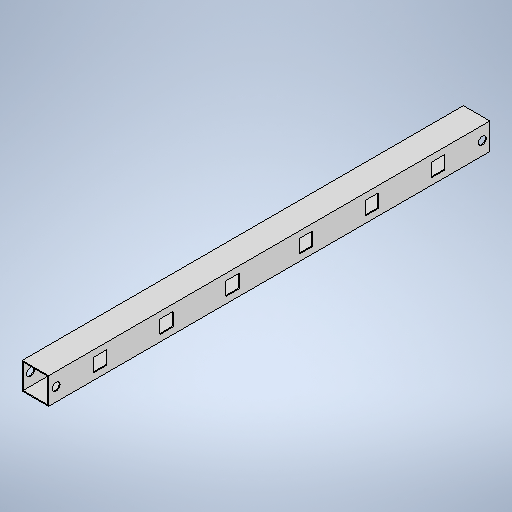
# Autodesk Inventor part: TZS 1761 FDS 1200x50 central way
Saved by Autodesk Inventor 2025.1 (Build 291241020, 241B)
## iProperties
Created: 2025-06-24
Part Number: TZS 1761 FDS 1200x50 central way
Material: Stainless Steel
Document SubType Name: Modeling
Designer: user
Mass: 1762.25 g
Surface Area: 2283.33 cm^2
Volume: 220.281 cm^3
Density: 8 g/cm^3
Sheet Metal Rule: AISI304 2mm Die16
Sheet Metal Width: 0.000 mm
Sheet Metal Length: 0.000 mm
Sheet Metal Area: 0.000 mm^2
Appearance: Default
Author: user
Autodesk Inventor part; units mm, degrees
ref_plane "YZ Plane" through (0, 0, 0) normal (1, 0, 0) x (0, 1, 0)
ref_plane "XZ Plane" through (0, 0, 0) normal (0, 1, 0) x (-1, 0, 0)
ref_plane "XY Plane" through (0, 0, 0) normal (0, 0, 1) x (1, 0, 0)
sketch "Sketch9" plane through (0, 0, 0) normal (0, 1, 0) x (-1, 0, 0)
  line L0 (30, 30) -> (-30, 30)
  line L1 (-30, 30) -> (-30, -30)
  line L2 (-30, -30) -> (30, -30)
  line L3 (30, -30) -> (30, 30)
  line L4 (30, 30) -> (-30, -30) construction
  line L5 (-30, 30) -> (30, -30) construction
  line L6 (-28, 28) -> (28, 28)
  line L7 (28, 28) -> (28, -28)
  line L8 (28, -28) -> (-28, -28)
  line L9 (-28, -28) -> (-28, 28)
  point P0 (0, 0)
  dimension "d172" = 60
  dimension "d173" = 60
  dimension "d174" = 2
  constraints: 20 end point, 4 parallel, 2 midpoint, 2 perpendicular, 1 horizontal, 3 other
  measures "d172" distance of L2.end L1.end
  measures "d173" distance of L0.end L1.end
  measures "d174" distance between parallel lines of L0 L6
extrude "Extrusion3" add sketch "Sketch9" against normal blind 500
sketch "Sketch10" plane through (0, 0, 0) normal (1, 0, 0) x (0, 1, 0)
  line L0 (0, 30) -> (0, -30) construction
  line L1 (0, 30) -> (-500, 30) construction
  line L2 (-500, -30) -> (-500, 30) construction
  line L3 (0, -30) -> (-500, -30) construction
  line L4 (-98.25, 15.25) -> (-67.75, 15.25)
  line L5 (-67.75, 15.25) -> (-67.75, -15.25)
  line L6 (-67.75, -15.25) -> (-98.25, -15.25)
  line L7 (-98.25, -15.25) -> (-98.25, 15.25)
  line L8 (-98.25, 15.25) -> (-67.75, -15.25) construction
  line L9 (-67.75, 15.25) -> (-98.25, -15.25) construction
  line L10 (-248.25, 15.25) -> (-217.75, 15.25)
  line L11 (-217.75, 15.25) -> (-217.75, -15.25)
  line L12 (-217.75, -15.25) -> (-248.25, -15.25)
  line L13 (-248.25, -15.25) -> (-248.25, 15.25)
  line L14 (-248.25, 15.25) -> (-217.75, -15.25) construction
  line L15 (-217.75, 15.25) -> (-248.25, -15.25) construction
  line L16 (-398.25, 15.25) -> (-367.75, 15.25)
  line L17 (-367.75, 15.25) -> (-367.75, -15.25)
  line L18 (-367.75, -15.25) -> (-398.25, -15.25)
  line L19 (-398.25, -15.25) -> (-398.25, 15.25)
  line L20 (-398.25, 15.25) -> (-367.75, -15.25) construction
  line L21 (-367.75, 15.25) -> (-398.25, -15.25) construction
  circle A0 centre (-483, 0) radius 9
  line L22 (0, 0) -> (47, 0)
  point P0 (-83, 0)
  point P1 (-233, 0)
  point P2 (-383, 0)
  dimension "d177" = 30.5
  dimension "d178" = 30.5
  dimension "d181" = 47
  dimension "d182" = 130
  dimension "d183" = 280
  dimension "d184" = 430
  dimension "d185" = 530
  dimension "d186" = 18
  constraints: 38 end point, 7 midpoint, 6 parallel, 4 horizontal, 4 horizontal alignment, 3 equal length, 3 perpendicular, 1 centre point, 1 point on line
  measures "d177" distance of L4.start L4.end
  measures "d178" distance of L4.end L5.end
  measures "d181" distance of L22.start L22.end
  measures "d182" distance of point (-83, 0) L22.end
  measures "d183" distance of point (-233, 0) L22.end
  measures "d184" distance of L22.end point (-383, 0)
  measures "d185" distance of L22.end A0.centre
  measures "d186" diameter of A0
extrude "Extrusion4" cut sketch "Sketch10" along normal through all both and the other way through all
fillet "Fillet1" radius 2 24 edges at (29, -367.75, -15.25) (29, -367.75, 15.25) (29, -398.25, 15.25) (29, -398.25, -15.25) (29, -248.25, -15.25) (29, -248.25, 15.25) (29, -217.75, 15.25) (29, -217.75, -15.25) (29, -98.25, 15.25) (29, -67.75, 15.25) (29, -67.75, -15.25) (29, -98.25, -15.25) (-29, -98.25, 15.25) (-29, -67.75, 15.25) (-29, -67.75, -15.25) (-29, -98.25, -15.25) (-29, -217.75, 15.25) (-29, -248.25, 15.25) (-29, -248.25, -15.25) (-29, -217.75, -15.25) (-29, -367.75, 15.25) (-29, -398.25, 15.25) (-29, -367.75, -15.25) (-29, -398.25, -15.25)
mirror "Mirror1" about plane through (0, 0, 0) normal (0, 1, 0) of "Extrusion3", "Extrusion4", "Fillet1"
sketch "Sketch14" plane through (30, -500, -30) normal (0, 0, -1) x (-1, 0, 0)
  line L0 (57, 527) -> (3, 527)
  line L1 (3, 527) -> (3, 473)
  line L2 (3, 473) -> (57, 473)
  line L3 (57, 473) -> (57, 527)
  line L4 (57, 527) -> (3, 473) construction
  line L5 (3, 527) -> (57, 473) construction
  point P0 (30, 500)
  dimension "d188" = 54
  constraints: 12 end point, 2 midpoint, 2 parallel, 2 perpendicular, 1 horizontal
  measures "d188" distance of L2.end L1.end
extrude "Extrusion5" cut sketch "Sketch14" against normal up to surface (2 mm away)
fillet "Fillet2" radius 2 4 edges at (-27, -27, -29) (-27, 27, -29) (27, -27, -29) (27, 27, -29)
sketch "Sketch15" plane through (30, -500, 30) normal (1, 0, 0) x (0, 0, -1)
  line L0 (43.25, 717.75) -> (16.75, 717.75) projected
  arc A0 (14.75, 719.75) -> (16.75, 717.75) centre (16.75, 719.75) ccw projected
  line L1 (14.75, 719.75) -> (14.75, 746.25) projected
  arc A1 (16.75, 748.25) -> (14.75, 746.25) centre (16.75, 746.25) ccw projected
  line L2 (16.75, 748.25) -> (43.25, 748.25) projected
  arc A2 (45.25, 746.25) -> (43.25, 748.25) centre (43.25, 746.25) ccw projected
  line L3 (45.25, 746.25) -> (45.25, 719.75) projected
  arc A3 (43.25, 717.75) -> (45.25, 719.75) centre (43.25, 719.75) ccw projected
  line L4 (16.75, 898.25) -> (43.25, 898.25) projected
  arc A4 (45.25, 896.25) -> (43.25, 898.25) centre (43.25, 896.25) ccw projected
  line L5 (45.25, 896.25) -> (45.25, 869.75) projected
  arc A5 (43.25, 867.75) -> (45.25, 869.75) centre (43.25, 869.75) ccw projected
  line L6 (43.25, 867.75) -> (16.75, 867.75) projected
  arc A6 (14.75, 869.75) -> (16.75, 867.75) centre (16.75, 869.75) ccw projected
  line L7 (14.75, 869.75) -> (14.75, 896.25) projected
  arc A7 (16.75, 898.25) -> (14.75, 896.25) centre (16.75, 896.25) ccw projected
  line L8 (16.75, 598.25) -> (43.25, 598.25) projected
  arc A8 (45.25, 596.25) -> (43.25, 598.25) centre (43.25, 596.25) ccw projected
  line L9 (45.25, 596.25) -> (45.25, 569.75) projected
  arc A9 (43.25, 567.75) -> (45.25, 569.75) centre (43.25, 569.75) ccw projected
  line L10 (43.25, 567.75) -> (16.75, 567.75) projected
  arc A10 (14.75, 569.75) -> (16.75, 567.75) centre (16.75, 569.75) ccw projected
  line L11 (14.75, 569.75) -> (14.75, 596.25) projected
  arc A11 (16.75, 598.25) -> (14.75, 596.25) centre (16.75, 596.25) ccw projected
  circle A12 centre (30, 983) radius 9 projected
  line L12 (43.25, 251.75) -> (16.75, 251.75) projected
  arc A13 (14.75, 253.75) -> (16.75, 251.75) centre (16.75, 253.75) ccw projected
  line L13 (14.75, 253.75) -> (14.75, 280.25) projected
  arc A14 (16.75, 282.25) -> (14.75, 280.25) centre (16.75, 280.25) ccw projected
  line L14 (16.75, 282.25) -> (43.25, 282.25) projected
  arc A15 (45.25, 280.25) -> (43.25, 282.25) centre (43.25, 280.25) ccw projected
  line L15 (45.25, 280.25) -> (45.25, 253.75) projected
  arc A16 (43.25, 251.75) -> (45.25, 253.75) centre (43.25, 253.75) ccw projected
  circle A17 centre (30, 17) radius 9 projected
  line L16 (43.25, 401.75) -> (16.75, 401.75) projected
  arc A18 (14.75, 403.75) -> (16.75, 401.75) centre (16.75, 403.75) ccw projected
  line L17 (14.75, 403.75) -> (14.75, 430.25) projected
  arc A19 (16.75, 432.25) -> (14.75, 430.25) centre (16.75, 430.25) ccw projected
  line L18 (16.75, 432.25) -> (43.25, 432.25) projected
  arc A20 (45.25, 430.25) -> (43.25, 432.25) centre (43.25, 430.25) ccw projected
  line L19 (45.25, 430.25) -> (45.25, 403.75) projected
  arc A21 (43.25, 401.75) -> (45.25, 403.75) centre (43.25, 403.75) ccw projected
  line L20 (43.25, 101.75) -> (16.75, 101.75) projected
  arc A22 (14.75, 103.75) -> (16.75, 101.75) centre (16.75, 103.75) ccw projected
  line L21 (14.75, 103.75) -> (14.75, 130.25) projected
  arc A23 (16.75, 132.25) -> (14.75, 130.25) centre (16.75, 130.25) ccw projected
  line L22 (16.75, 132.25) -> (43.25, 132.25) projected
  arc A24 (45.25, 130.25) -> (43.25, 132.25) centre (43.25, 130.25) ccw projected
  line L23 (45.25, 130.25) -> (45.25, 103.75) projected
  arc A25 (43.25, 101.75) -> (45.25, 103.75) centre (43.25, 103.75) ccw projected
  line L24 (0, 1000) -> (0, 0) projected
  line L25 (60, 0) -> (0, 0) projected
  line L26 (60, 0) -> (60, 1000) projected
  line L27 (60, 1000) -> (0, 1000) projected
  line L28 (16.75, 130.25) -> (43.25, 103.75)
  line L29 (16.75, 280.25) -> (43.25, 253.75)
  line L30 (16.75, 430.25) -> (43.25, 403.75)
  line L31 (16.75, 596.25) -> (43.25, 569.75)
  line L32 (16.75, 746.25) -> (43.25, 719.75)
  line L33 (16.75, 896.25) -> (43.25, 869.75)
  point P0 (30, 500)
  constraints: 12 end point
sketch "Sketch16" plane through (-30, -500, -30) normal (-1, 0, 0) x (0, 0, 1)
  line L0 (45.25, 896.25) -> (45.25, 869.75) projected
  arc A0 (43.25, 867.75) -> (45.25, 869.75) centre (43.25, 869.75) ccw projected
  line L1 (43.25, 867.75) -> (16.75, 867.75) projected
  arc A1 (14.75, 869.75) -> (16.75, 867.75) centre (16.75, 869.75) ccw projected
  line L2 (14.75, 869.75) -> (14.75, 896.25) projected
  arc A2 (16.75, 898.25) -> (14.75, 896.25) centre (16.75, 896.25) ccw projected
  line L3 (16.75, 898.25) -> (43.25, 898.25) projected
  arc A3 (45.25, 896.25) -> (43.25, 898.25) centre (43.25, 896.25) ccw projected
  line L4 (43.25, 567.75) -> (16.75, 567.75) projected
  arc A4 (14.75, 569.75) -> (16.75, 567.75) centre (16.75, 569.75) ccw projected
  line L5 (14.75, 569.75) -> (14.75, 596.25) projected
  arc A5 (16.75, 598.25) -> (14.75, 596.25) centre (16.75, 596.25) ccw projected
  line L6 (16.75, 598.25) -> (43.25, 598.25) projected
  arc A6 (45.25, 596.25) -> (43.25, 598.25) centre (43.25, 596.25) ccw projected
  line L7 (45.25, 596.25) -> (45.25, 569.75) projected
  arc A7 (43.25, 567.75) -> (45.25, 569.75) centre (43.25, 569.75) ccw projected
  circle A8 centre (30, 983) radius 9 projected
  line L8 (43.25, 717.75) -> (16.75, 717.75) projected
  arc A9 (14.75, 719.75) -> (16.75, 717.75) centre (16.75, 719.75) ccw projected
  line L9 (14.75, 719.75) -> (14.75, 746.25) projected
  arc A10 (16.75, 748.25) -> (14.75, 746.25) centre (16.75, 746.25) ccw projected
  line L10 (16.75, 748.25) -> (43.25, 748.25) projected
  arc A11 (45.25, 746.25) -> (43.25, 748.25) centre (43.25, 746.25) ccw projected
  line L11 (45.25, 746.25) -> (45.25, 719.75) projected
  arc A12 (43.25, 717.75) -> (45.25, 719.75) centre (43.25, 719.75) ccw projected
  line L12 (43.25, 251.75) -> (16.75, 251.75) projected
  arc A13 (14.75, 253.75) -> (16.75, 251.75) centre (16.75, 253.75) ccw projected
  line L13 (14.75, 253.75) -> (14.75, 280.25) projected
  arc A14 (16.75, 282.25) -> (14.75, 280.25) centre (16.75, 280.25) ccw projected
  line L14 (16.75, 282.25) -> (43.25, 282.25) projected
  arc A15 (45.25, 280.25) -> (43.25, 282.25) centre (43.25, 280.25) ccw projected
  line L15 (45.25, 280.25) -> (45.25, 253.75) projected
  arc A16 (43.25, 251.75) -> (45.25, 253.75) centre (43.25, 253.75) ccw projected
  circle A17 centre (30, 17) radius 9 projected
  line L16 (43.25, 401.75) -> (16.75, 401.75) projected
  arc A18 (14.75, 403.75) -> (16.75, 401.75) centre (16.75, 403.75) ccw projected
  line L17 (14.75, 403.75) -> (14.75, 430.25) projected
  arc A19 (16.75, 432.25) -> (14.75, 430.25) centre (16.75, 430.25) ccw projected
  line L18 (16.75, 432.25) -> (43.25, 432.25) projected
  arc A20 (45.25, 430.25) -> (43.25, 432.25) centre (43.25, 430.25) ccw projected
  line L19 (45.25, 430.25) -> (45.25, 403.75) projected
  arc A21 (43.25, 401.75) -> (45.25, 403.75) centre (43.25, 403.75) ccw projected
  line L20 (43.25, 101.75) -> (16.75, 101.75) projected
  arc A22 (14.75, 103.75) -> (16.75, 101.75) centre (16.75, 103.75) ccw projected
  line L21 (14.75, 103.75) -> (14.75, 130.25) projected
  arc A23 (16.75, 132.25) -> (14.75, 130.25) centre (16.75, 130.25) ccw projected
  line L22 (16.75, 132.25) -> (43.25, 132.25) projected
  arc A24 (45.25, 130.25) -> (43.25, 132.25) centre (43.25, 130.25) ccw projected
  line L23 (45.25, 130.25) -> (45.25, 103.75) projected
  arc A25 (43.25, 101.75) -> (45.25, 103.75) centre (43.25, 103.75) ccw projected
  line L24 (0, 0) -> (0, 1000) projected
  line L25 (60, 0) -> (0, 0) projected
  line L26 (60, 0) -> (60, 1000) projected
  line L27 (60, 1000) -> (0, 1000) projected
  line L28 (43.25, 869.75) -> (16.75, 896.25)
  line L29 (43.25, 719.75) -> (16.75, 746.25)
  line L30 (43.25, 569.75) -> (16.75, 596.25)
  line L31 (43.25, 403.75) -> (16.75, 430.25)
  line L32 (43.25, 253.75) -> (16.75, 280.25)
  arc A26 (16.75, 132.25) -> (14.75, 130.25) centre (16.75, 130.25) ccw projected
  line L33 (43.25, 103.75) -> (16.75, 130.25)
  point P0 (30, 500)
  constraints: 12 end point, 2 coincident
body "Solid4"
